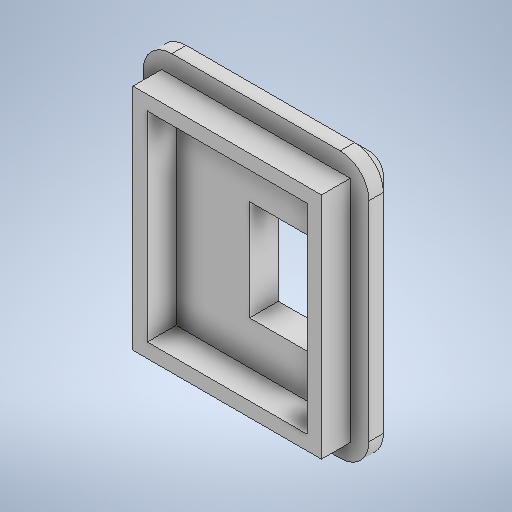
# Autodesk Inventor part: VL53L0X_cover_2
Saved by Autodesk Inventor 2025.3 (Build 293356000, 356)
## iProperties
Created: 2025-11-14
Part Number: VL53L0X_cover_2
Material: Generic
Document SubType Name: Modeling
Designer: woyao
Density: 1 g/cm^3
Appearance: Default
Author: woyao
Autodesk Inventor part; units mm, degrees
ref_plane "YZ Plane" through (0, 0, 0) normal (1, 0, 0) x (0, 1, 0)
ref_plane "XZ Plane" through (0, 0, 0) normal (0, 1, 0) x (-1, 0, 0)
ref_plane "XY Plane" through (0, 0, 0) normal (0, 0, 1) x (1, 0, 0)
sketch "Sketch1" plane through (0, 0, 0) normal (0, 0, 1) x (1, 0, 0)
  point P0 (0, 0)
sketch "Sketch2" plane through (0, 0, 0) normal (0, 0, 1) x (1, 0, 0)
  point P0 (0, 0)
sketch "Sketch3" plane through (0, 0, 0) normal (0, 0, 1) x (1, 0, 0)
  line L0 (0, 0) -> (11.1, 0)
  line L1 (11.1, 0) -> (11.1, 13.9)
  line L2 (11.1, 13.9) -> (0, 13.9)
  line L3 (0, 13.9) -> (0, 0)
  line L4 (-1, -1) -> (12.1, -1)
  line L5 (12.1, -1) -> (12.1, 14.9)
  line L6 (12.1, 14.9) -> (-1, 14.9)
  line L7 (-1, 14.9) -> (-1, -1)
  dimension "d0" = 13.9
  dimension "d1" = 11.1
  dimension "d7" = 1
  constraints: 16 end point, 4 parallel, 2 perpendicular, 1 horizontal, 3 other
  measures "d0" distance of L2.end L0.start
  measures "d1" distance of L0.start L0.end
  measures "d7" distance between parallel lines of L3 L7
extrude "Extrusion1" add sketch "Sketch3" along normal blind 2
sketch "Sketch5" plane through (0, 0, 0) normal (0, 0, -1) x (-1, 0, 0)
  line L0 (-12.1, 14.9) -> (1, 14.9) projected
  line L1 (-12.1, -1) -> (-12.1, 14.9) projected
  line L2 (1, 14.9) -> (1, -1) projected
  line L3 (1, -1) -> (-12.1, -1) projected
  line L4 (2.3, 16.2) -> (-13.4, 16.2)
  line L5 (-13.4, 16.2) -> (-13.4, -2.3)
  line L6 (-13.4, -2.3) -> (2.3, -2.3)
  line L7 (2.3, -2.3) -> (2.3, 16.2)
  point P0 (0, 0)
  dimension "d8" = 1.3
  constraints: 8 end point, 3 other
  measures "d8" distance between parallel lines of L0 L4
extrude "Extrusion2" add sketch "Sketch5" along normal blind 2 contours L0 L2 L3 L1 | L7 L6 L5 L4
sketch "Sketch7" plane through (0, 0, 0) normal (0, 0, 1) x (1, 0, 0)
  line L0 (5.1, 3) -> (11.1, 3)
  line L1 (11.1, 3) -> (11.1, 10)
  line L2 (11.1, 10) -> (5.1, 10)
  line L3 (5.1, 10) -> (5.1, 3)
  line L4 (0, 0) -> (0, 13.9) projected
  line L5 (11.1, 0) -> (0, 0) projected
  line L6 (11.1, 13.9) -> (11.1, 0) projected
  dimension "d16" = 7
  dimension "d17" = 6
  dimension "d22" = 3
  dimension "d23" = 0
  constraints: 8 end point, 2 parallel, 1 horizontal, 1 perpendicular
  measures "d16" distance of L2.end L0.start
  measures "d17" distance of L0.start L0.end
  measures "d22" distance between parallel lines of L5 L0
  measures "d23" distance between parallel lines of L6 L1
extrude "Extrusion4" cut sketch "Sketch7" against normal blind 2
fillet "Fillet1" radius 2 4 edges at (13.4, 16.2, -1) (-2.3, 16.2, -1) (13.4, -2.3, -1) (-2.3, -2.3, -1)
chamfer "Chamfer1" distance 1 angle 45 8 edges at (5.55, 16.2, -2) (12.8142, 15.6142, -2) (13.4, 6.95, -2) (12.8142, -1.7142, -2) (5.55, -2.3, -2) (-1.7142, -1.7142, -2) (-2.3, 6.95, -2) (-1.7142, 15.6142, -2)
body "Solid1"
